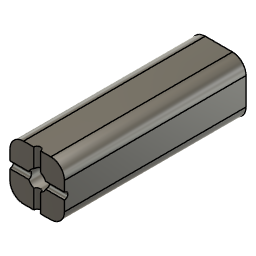
2024-10-04-wire-strip-jig (Autodesk Fusion 360 design; units mm, degrees)
Autodesk Fusion 360 part; units mm, degrees
sketch "Sketch1" plane through (0, 0, 0) normal (0, 0, 1) x (1, 0, 0)
  line L0 (-7.62, 3.81) -> (-7.62, -3.81)
  line L1 (-3.81, -7.62) -> (3.81, -7.62)
  line L2 (7.62, -3.81) -> (7.62, 3.81)
  line L3 (3.81, 7.62) -> (-3.81, 7.62)
  line L4 (-7.62, 7.62) -> (7.62, -7.62) construction
  line L5 (7.62, 7.62) -> (-7.62, -7.62) construction
  circle A0 centre (0, 0) radius 2.54
  arc A1 (-3.81, 7.62) -> (-7.62, 3.81) centre (-3.81, 3.81) ccw
  arc A2 (-7.62, -3.81) -> (-3.81, -7.62) centre (-3.81, -3.81) ccw
  arc A3 (7.62, 3.81) -> (3.81, 7.62) centre (3.81, 3.81) ccw
  arc A4 (3.81, -7.62) -> (7.62, -3.81) centre (3.81, -3.81) ccw
  dimension "d1" = 5.08
  dimension "d2" = 3.81
  dimension "d3" = 7.62
  dimension "d5" = 3.81
  dimension "d6" = 3.81
  dimension "d7" = 3.81
  constraint vertical L0
  constraint perpendicular L0 L1
  constraint perpendicular L1 L2
  constraint perpendicular L0 L3
  constraint perpendicular L4 L5
  constraint midpoint L5 A0.centre
  constraint coincident L4.start L3
  constraint coincident L4.start L0
  constraint tangent L3 A1
  constraint tangent L0 A1
  constraint coincident L5.end L0
  constraint coincident L5.end L1
  constraint tangent L0 A2
  constraint tangent L1 A2
  constraint coincident L5.start L3
  constraint coincident L5.start L2
  constraint tangent L3 A3
  constraint tangent L2 A3
  constraint coincident L4.end L2
  constraint coincident L4.end L1
  constraint tangent L2 A4
  constraint tangent L1 A4
  constraint coincident A0.centre origin
  measures "d1" diameter of A0
  measures "d2" radius of A1
  measures "d3" distance of L0 A0.centre
  measures "d5" radius of A2
  measures "d6" radius of A3
  measures "d7" radius of A4
extrude "Extrude1" add sketch "Sketch1" against normal blind 50.8
sketch "Sketch2" plane through (0, 7.62, 0) normal (0, 1, 0) x (-1, 0, 0)
  line L0 (3.81, 0) -> (-3.81, 0)
  line L1 (3.81, -50.8) -> (3.81, 0)
  line L2 (-3.81, -50.8) -> (3.81, -50.8)
  line L3 (-3.81, 0) -> (-3.81, -50.8)
  circle A0 centre (0, 0) radius 0.9525
  dimension "d11" = 1.905
  constraint coincident A0.centre origin
  measures "d11" diameter of A0
extrude "Extrude2" cut sketch "Sketch2" against normal through all contours L0 A0 picked at (-0.2327, -0.216)
sketch "Sketch3" plane through (-7.62, 0, 0) normal (-1, 0, 0) x (0, 0, 1)
  line L0 (0, -3.81) -> (0, 3.81)
  line L1 (-50.8, -3.81) -> (0, -3.81)
  line L2 (-50.8, 3.81) -> (-50.8, -3.81)
  line L3 (0, 3.81) -> (-50.8, 3.81)
  circle A0 centre (0, 0) radius 0.9525
  dimension "d13" = 1.905
  constraint coincident A0.centre origin
  measures "d13" diameter of A0
extrude "Extrude3" cut sketch "Sketch3" against normal through all contours L0 A0 picked at (-0.1378, -0.2861)
equation "d2 = d3 / 2"
equation "d3 = d1 / 2 + WireInsulationLength"
equation "WireInsulationLength = 0.2 in"
equation "d5 = d3 / 2"
equation "d6 = d3 / 2"
equation "d7 = d3 / 2"
equation "d8 = -2\""
equation "WireChannelDiameter = 0.075 in"
equation "d11 = WireChannelDiameter"
equation "d13 = WireChannelDiameter"
named bodies: "wire-strip-jig"
